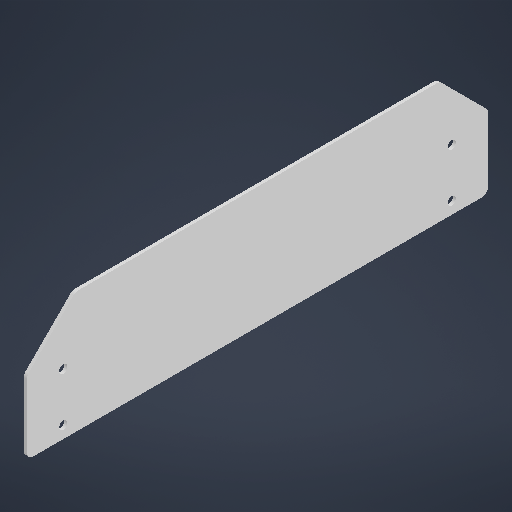
# Autodesk Inventor part: wedge
Saved by Autodesk Inventor 2025.2 (Build 292293000, 293)
## iProperties
Created: 2025-03-30
Part Number: wedge
Material: Generic
Document SubType Name: Modeling
Designer: roejo
Density: 1 g/cm^3
Appearance: Default
Author: roejo
Autodesk Inventor part; units mm, degrees
ref_plane "YZ Plane" through (0, 0, 0) normal (1, 0, 0) x (0, 1, 0)
ref_plane "XZ Plane" through (0, 0, 0) normal (0, 1, 0) x (-1, 0, 0)
ref_plane "XY Plane" through (0, 0, 0) normal (0, 0, 1) x (1, 0, 0)
sketch "Sketch1" plane through (0, 0, 0) normal (1, 0, 0) x (0, 1, 0)
  line L0 (-31.0872, -5.216) -> (-31.0872, 56.252)
  line L1 (-31.0872, -117.4332) -> (-31.0872, 117.5168)
  line L2 (-27.9122, 120.6918) -> (5.6976, 120.6918)
  line L3 (-27.9122, -120.6082) -> (5.6976, -120.6082)
  line L4 (32.4128, 93.9766) -> (32.4128, -93.8931)
  line L5 (7.9427, 119.7618) -> (31.4828, 96.2217)
  line L6 (7.9427, -119.6783) -> (31.4828, -96.1382)
  arc A0 (32.4128, 93.9766) -> (31.4828, 96.2217) centre (29.2378, 93.9766) ccw
  arc A1 (31.4828, -96.1382) -> (32.4128, -93.8931) centre (29.2378, -93.8931) ccw
  arc A2 (5.6976, -120.6082) -> (7.9427, -119.6783) centre (5.6976, -117.4332) ccw
  arc A3 (-31.0872, -117.4332) -> (-27.9122, -120.6082) centre (-27.9122, -117.4332) ccw
  arc A4 (-27.9122, 120.6918) -> (-31.0872, 117.5168) centre (-27.9122, 117.5168) ccw
  arc A5 (7.9427, 119.7618) -> (5.6976, 120.6918) centre (5.6976, 117.5168) ccw
  circle A6 centre (0.6628, 101.6418) radius 2.1844
  circle A7 centre (-24.7372, 101.6418) radius 2.1844
  circle A8 centre (-24.7372, -101.5582) radius 2.1844
  circle A9 centre (0.6628, -101.5582) radius 2.1844
  point P0 (0, 0)
  point P1 (-31.0872, -120.6082)
  point P2 (-31.0872, 120.6918)
  point P3 (7.0128, 120.6918)
  point P4 (7.0128, -120.6082)
  dimension "d0" = 241.3
  dimension "d1" = 38.1
  dimension "d2" = 38.1
  dimension "d3" = 3.175
  dimension "d4" = 3.175
  dimension "d5" = 3.175
  dimension "d6" = 3.175
  dimension "d7" = 3.175
  dimension "d8" = 3.175
  dimension "d15" = 4.3688
  dimension "d16" = 4.3688
  dimension "d17" = 4.3688
  dimension "d18" = 4.3688
  constraints: 14 end point, 12 point on circle, 12 tangent, 10 centre point, 10 point on line, 2 perpendicular, 1 horizontal
  measures "d0" distance of point (-31.087, -120.608) point (-31.087, 120.692)
  measures "d1" distance of point (-31.087, 120.692) point (7.013, 120.692)
  measures "d2" distance of point (-31.087, -120.608) point (7.013, -120.608)
  measures "d3" radius of A0
  measures "d4" radius of A1
  measures "d5" radius of A2
  measures "d6" radius of A3
  measures "d7" radius of A4
  measures "d8" radius of A5
  measures "d15" diameter of A6
  measures "d16" diameter of A7
  measures "d17" diameter of A8
  measures "d18" diameter of A9
extrude "Extrusion1" add sketch "Sketch1" along normal blind 1.5875
body "Solid1"
